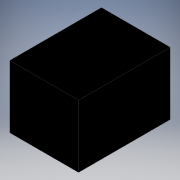
# Autodesk Inventor part: Computer
Saved by Autodesk Inventor 2017 (Build 210142000, 142)
## iProperties
Created: 2017-02-10
Part Number: Computer
Material: Generic
Document SubType Name: Modeling
Designer: michael
Density: 1 g/cm^3
Appearance: Default
Author: michael
Autodesk Inventor part; units mm, degrees
ref_plane "YZ Plane" through (0, 0, 0) normal (1, 0, 0) x (0, 1, 0)
ref_plane "XZ Plane" through (0, 0, 0) normal (0, 1, 0) x (-1, 0, 0)
ref_plane "XY Plane" through (0, 0, 0) normal (0, 0, 1) x (1, 0, 0)
sketch "Sketch1" plane through (0, 0, 0) normal (0, 1, 0) x (-1, 0, 0)
  line L0 (-104.775, 139.7) -> (104.775, 139.7)
  line L1 (104.775, 139.7) -> (104.775, -139.7)
  line L2 (104.775, -139.7) -> (-104.775, -139.7)
  line L3 (-104.775, -139.7) -> (-104.775, 139.7)
  line L4 (-104.775, 139.7) -> (104.775, -139.7) construction
  line L5 (104.775, 139.7) -> (-104.775, -139.7) construction
  point P0 (0, 0)
  dimension "d0" = 209.55
  dimension "d1" = 279.4
  constraints: 12 end point, 2 midpoint, 2 parallel, 1 horizontal, 1 perpendicular
  measures "d0" distance of L1.end L2.end
  measures "d1" distance of L0.end L1.end
extrude "Extrusion1" add sketch "Sketch1" along normal blind 190.5
body "Solid1"
